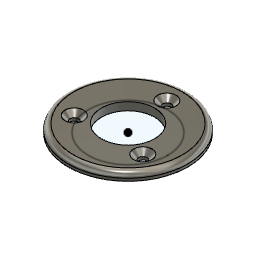
Paddle Mount Rotary Encoder v2 (Autodesk Fusion 360 design; units mm, degrees)
Autodesk Fusion 360 part; units mm, degrees
sketch "Sketch1" plane through (0, 0, 0) normal (0, 1, 0) x (1, 0, 0)
  circle A0 centre (0, 0) radius 22.661
  constraint coincident A0.centre origin
extrude "Extrude1" add sketch "Sketch1" along normal blind 3
hole "Hole1" at (0, 3, 0) direction (0, -1, 0) diameter 20.2 depth 3 tip angle 180
hole "Hole2" at (-0.1263, 3, -14.8781) direction (0, -1, 0) diameter 3.2 depth 30 tip angle 180 countersink diameter 7 countersink angle 90
sketch "Sketch2" plane through (0, 0, 0) normal (0, 1, 0) x (1, 0, 0)
  circle A0 centre (0, 0) radius 15
  dimension "d9" = 30
  constraint coincident A0.centre origin
  measures "d9" diameter of A0
pattern_circular "C-Pattern1" count 3 over 360 about axis through (0, 0, 0) along (0, 1, 0) of "Hole2"
fillet "Fillet1" radius 2 1 edges at (-21.1274, 3, 8.1946)
